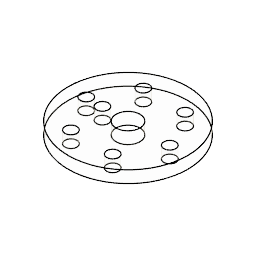
LowerVertibraeV1_v3 (Autodesk Fusion 360 design; units mm, degrees)
Autodesk Fusion 360 part; units mm, degrees
sketch "Sketch1" plane through (0, 0, 0) normal (0, 0, 1) x (1, 0, 0)
  circle A0 centre (0, 0) radius 10
  circle A1 centre (0, 0) radius 2
  circle A2 centre (-7, 0) radius 1
  line L0 (0, 0) -> (-7, 0) construction
  circle A3 centre (-3.5, -6.0622) radius 1
  line L1 (0, 0) -> (-3.5, -6.0622) construction
  circle A4 centre (3.5, -6.0622) radius 1
  line L2 (0, 0) -> (3.5, -6.0622) construction
  circle A5 centre (7, 0) radius 1
  line L3 (0, 0) -> (7, 0) construction
  circle A6 centre (3.5, 6.0622) radius 1
  line L4 (0, 0) -> (3.5, 6.0622) construction
  circle A7 centre (-3.5, 6.0622) radius 1
  line L5 (0, 0) -> (-3.5, 6.0622) construction
  line L6 (0, 0) -> (-3, 0)
  line L7 (0, 0) -> (1.7321, 1) construction
  line L8 (0, 0) -> (-1.7321, -1) construction
  line L9 (1.7321, 1) -> (3.0311, 1.75) construction
  circle A8 centre (-4.2794, -0.0013) radius 1
  line L10 (-4.2794, -0.0013) -> (0, 0) construction
  dimension "d1" = 20
  dimension "d4" = 4
  dimension "d7" = 2
  dimension "d8" = 7
  dimension "d10" = 360
  dimension "d18" = 2
  constraint coincident A0.centre A1.centre
  constraint coincident A2.centre L0.end
  constraint horizontal L0
  constraint coincident L0 L6.end
  constraint coincident A1 L7.end
  constraint coincident A1 L8.end
  constraint coincident A8.centre L10.start
  measures "d1" diameter of A0
  measures "d4" diameter of A1
  measures "d7" diameter of A2
  measures "d8" distance of A0.centre A2.centre
  measures "d18" diameter of A8
extrude "Extrude1" add sketch "Sketch1" along normal blind 2
